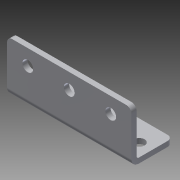
# Autodesk Inventor part: Chassis Bumper Mount - side - center
Saved by Autodesk Inventor 2013 (Build 170138000, 138)
## iProperties
Created: 2013-01-25
Part Number: Chassis Bumper Mount - side - center
Material: Aluminum 6061
Document SubType Name: Sheet Metal
Designer: Moses
Mass: 33.0362 g
Surface Area: 88.0991 cm^2
Volume: 12.1905 cm^3
Density: 2.71 g/cm^3
Flat Pattern Width: 5.24493 cm
Flat Pattern Length: 7.62 cm
Flat Pattern Area: 39.9664 cm^2
Sheet Metal Rule: Default
Sheet Metal Width: 2.065 in
Sheet Metal Length: 3.000 in
Sheet Metal Area: 6.195 in^2
Author: Moses
Autodesk Inventor part; units mm, degrees
ref_plane "YZ Plane" through (0, 0, 0) normal (1, 0, 0) x (0, 1, 0)
ref_plane "XZ Plane" through (0, 0, 0) normal (0, 1, 0) x (-1, 0, 0)
ref_plane "XY Plane" through (0, 0, 0) normal (0, 0, 1) x (1, 0, 0)
sketch "Sketch1" plane through (0, 0, 0) normal (0, 1, 0) x (-1, 0, 0)
  line L0 (0, 0) -> (76.2, 0)
  line L1 (76.2, 0) -> (76.2, 25.4)
  line L2 (76.2, 25.4) -> (0, 25.4)
  line L3 (0, 25.4) -> (0, 0)
  circle A0 centre (7.9375, 12.7) radius 3.302
  circle A1 centre (68.2625, 12.7) radius 3.302
  line L4 (7.9375, 12.7) -> (68.2625, 12.7) construction
  line L5 (38.1, 25.4) -> (38.1, 0) construction
  point P0 (38.1, 12.7)
  dimension "d0" = 76.2
  dimension "d1" = 25.4
  dimension "d2" = 6.604
  dimension "d3" = 60.325
  measures "d0" distance of L0.start L0.end
  measures "d1" distance of L2.end L0.start
  measures "d2" diameter of A0
  measures "d3" distance of L4.start L4.end
extrude "Plate1" add sketch "Sketch1" along normal blind 3.175
sketch "Sketch2" plane through (0, 0, 22.225) normal (0, 0, 1) x (1, 0, 0)
  line L0 (-76.2, 0) -> (0, 0)
  line L1 (0, 0) -> (0, 31.75)
  line L2 (0, 31.75) -> (-76.2, 31.75)
  line L3 (-76.2, 31.75) -> (-76.2, 0)
  constraints: 6 end point, 1 horizontal, 1 perpendicular, 1 vertical
edge flange "Flange1" height 31.75 angle 90 thickness 3.175 bend radius 1.27 thickness toward (0, 0, 1) relief straight relief width 3.175 relief depth 1.5875 edges at (-38.1, 3.175, 25.4) wall of the first edge with corners at (-76.2, 0, 22.225) (0, 0, 22.225) (0, 31.75, 22.225) (-76.2, 31.75, 22.225)
bend "Bend1"
corner "Corner1"
sketch "Sketch3" plane through (-76.2, 31.75, 25.4) normal (0, 0, 1) x (1, 0, 0)
  line L0 (0, -27.305) -> (76.2, -27.305) projected
  line L1 (0, 0) -> (76.2, 0) projected
  line L2 (0, -27.305) -> (0, 0) projected
  circle A0 centre (12.7, -9.525) radius 3.302
  circle A1 centre (38.1, -9.525) radius 3.302
  circle A2 centre (63.5, -9.525) radius 3.302
  line L3 (12.7, -9.525) -> (63.5, -9.525) construction
  line L4 (38.1, 0) -> (38.1, -38.1) construction
  line L5 (76.2, -31.75) -> (0, -31.75) projected
  dimension "d15" = 50.8
  dimension "d17" = 6.604
  dimension "d19" = 22.225
  constraints: 4 end point, 3 centre point, 2 equal radius, 2 midpoint, 2 perpendicular, 1 coincident, 1 point on line
  measures "d15" distance of L3.start L3.end
  measures "d17" diameter of A0
  measures "d19" distance between parallel lines of L5 L3
extrude "Cut1" cut sketch "Sketch3" against normal blind 3.175
fillet "Corner Round1" radius 3.175 4 edges at (0, 31.75, 23.8125) (-76.2, 31.75, 23.8125) (-76.2, 1.5875, 0) (0, 1.5875, 0)
equation "\"d20\" = Thickness"
equation "\"d5\" = BendReliefWidth"
equation "\"d6\" = BendReliefDepth"
equation "\"d7\" = MinimumRemnant"
equation "\"d8\" = BendRadius"
equation "\"d12\" = CornerReliefSize"
equation "\"d13\" = GapSize"
equation "\"d14\" = JacobiRadiusSize"
equation "\"BendRadius\" = Thickness"
equation "\"BendReliefWidth\" = Thickness"
equation "\"BendReliefDepth\" = 0.5 * Thickness"
equation "\"CornerReliefSize\" = 4 * Thickness"
equation "\"MinimumRemnant\" = 2 * Thickness"
equation "\"TransitionRadius\" = BendRadius"
equation "\"JacobiRadiusSize\" = BendRadius"
equation "\"GapSize\" = Thickness"
equation "\"d4\" = BendRadius"
equation "\"Thickness\" = 3.175"
body "Solid1"
